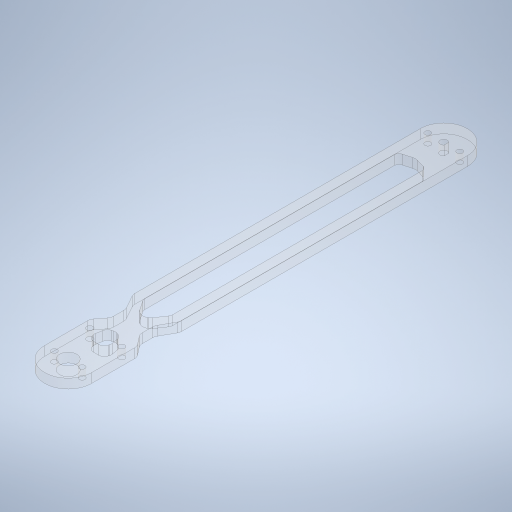
# Autodesk Inventor part: Part51
Saved by Autodesk Inventor 2024 (Build 280153000, 153)
## iProperties
Created: 2024-08-13
Part Number: Part51
Material: Polycarbonate, Clear
Document SubType Name: Modeling
Designer: David Ricaurte
Density: 1.2 g/cm^3
Appearance: Polycarbonate - Clear
Author: David Ricaurte
Autodesk Inventor part; units mm, degrees
ref_plane "YZ Plane" through (0, 0, 0) normal (1, 0, 0) x (0, 1, 0)
ref_plane "XZ Plane" through (0, 0, 0) normal (0, 1, 0) x (-1, 0, 0)
ref_plane "XY Plane" through (0, 0, 0) normal (0, 0, 1) x (1, 0, 0)
sketch "Sketch1" plane through (0, 0, 0) normal (0, 1, 0) x (-1, 0, 0)
  arc A0 (-1.4, -51.2845) -> (-1.4, -48.7155) centre (0, -50) ccw
  line L0 (-1.4, -48.7155) -> (-1.4, -51.2845)
  line L1 (-2.1842, 109.6159) -> (-1.9664, 109.7389)
  arc A1 (1.9664, 109.7389) -> (-1.9664, 109.7389) centre (0, 106.2556) ccw
  line L2 (1.9664, 109.7389) -> (2.1842, 109.6159)
  arc A2 (3.5277, 108.3788) -> (2.1842, 109.6159) centre (0.2179, 106.1326) ccw
  line L3 (3.5277, 108.3788) -> (8.2122, 101.4762)
  arc A3 (8.9023, 99.2105) -> (8.2122, 101.4762) centre (4.9024, 99.23) ccw
  line L4 (8.9023, 99.2105) -> (8.5178, 20.4265)
  arc A4 (5.6167, -33.4003) -> (8.5178, -29.5737) centre (4.5178, -29.5542) ccw
  line L5 (5.6167, -33.4003) -> (1.0989, -34.6911)
  arc A5 (-1.0989, -34.6911) -> (1.0989, -34.6911) centre (0, -30.845) ccw
  line L6 (-1.0989, -34.6911) -> (-5.6167, -33.4003)
  arc A6 (-8.5178, -29.5737) -> (-5.6167, -33.4003) centre (-4.5178, -29.5542) ccw
  line L7 (-8.5178, 20.4265) -> (-8.9023, 99.2105)
  arc A7 (-8.2122, 101.4762) -> (-8.9023, 99.2105) centre (-4.9024, 99.23) ccw
  line L8 (-8.2122, 101.4762) -> (-3.5277, 108.3788)
  arc A8 (-2.1842, 109.6159) -> (-3.5277, 108.3788) centre (-0.2179, 106.1326) ccw
  line L9 (-3.9333, 127.6797) -> (-4.4928, 131.0366)
  arc A9 (-4.4182, 132.354) -> (-4.4928, 131.0366) centre (-1.5336, 131.5298) ccw
  line L10 (-4.4182, 132.354) -> (-4.2433, 132.9662)
  arc A10 (-1.3587, 135.1421) -> (-4.2433, 132.9662) centre (-1.3587, 132.1421) ccw
  line L11 (-1.3587, 135.1421) -> (1.3587, 135.1421)
  arc A11 (4.2433, 132.9662) -> (1.3587, 135.1421) centre (1.3587, 132.1421) ccw
  line L12 (4.2433, 132.9662) -> (4.4182, 132.354)
  arc A12 (4.4928, 131.0366) -> (4.4182, 132.354) centre (1.5336, 131.5298) ccw
  line L13 (4.4928, 131.0366) -> (3.9333, 127.6797)
  arc A13 (1.7983, 125.2884) -> (3.9333, 127.6797) centre (0.9742, 128.1729) ccw
  line L14 (1.7983, 125.2884) -> (0.8242, 125.01)
  arc A14 (-0.8242, 125.01) -> (0.8242, 125.01) centre (0, 127.8946) ccw
  line L15 (-0.8242, 125.01) -> (-1.7983, 125.2884)
  arc A15 (-3.9333, 127.6797) -> (-1.7983, 125.2884) centre (-0.9742, 128.1729) ccw
  arc A16 (-12.5, 127.1805) -> (-11.6588, 124.7265) centre (-8.5, 127.1805) ccw
  line L16 (-11.6588, 124.7265) -> (-8.4827, 120.6384)
  arc A17 (-7.6415, 118.1843) -> (-8.4827, 120.6384) centre (-11.6415, 118.1843) ccw
  line L17 (-7.6415, 118.1843) -> (-7.6415, 112.7784)
  arc A18 (-8.147, 110.832) -> (-7.6415, 112.7784) centre (-11.6415, 112.7784) ccw
  line L18 (-8.147, 110.832) -> (-11.9945, 103.9244)
  arc A19 (-11.9945, 103.9244) -> (-12.5, 101.978) centre (-8.5, 101.978) ccw
  line L19 (-12.5, 101.978) -> (-12.5, 0)
  arc A20 (-12.5, -50) -> (12.5, -50) centre (0, -50) ccw
  line L20 (12.5, 0) -> (12.5, 101.978)
  arc A21 (12.5, 101.978) -> (11.9945, 103.9244) centre (8.5, 101.978) ccw
  line L21 (11.9945, 103.9244) -> (8.147, 110.832)
  arc A22 (7.6415, 112.7784) -> (8.147, 110.832) centre (11.6415, 112.7784) ccw
  line L22 (7.6415, 112.7784) -> (7.6415, 118.1843)
  arc A23 (8.4827, 120.6384) -> (7.6415, 118.1843) centre (11.6415, 118.1843) ccw
  line L23 (8.4827, 120.6384) -> (11.6588, 124.7265)
  arc A24 (11.6588, 124.7265) -> (12.5, 127.1805) centre (8.5, 127.1805) ccw
  line L24 (12.5, 127.1805) -> (12.5, 150)
  arc A25 (12.5, 150) -> (-12.5, 150) centre (0, 150) ccw
  line L25 (-12.5, 150) -> (-12.5, 127.1805)
  circle A26 centre (8.5, -50) radius 1.5
  circle A27 centre (-8.5, -50) radius 1.5
  circle A28 centre (0, 150) radius 4.5
  circle A29 centre (-8.5, 130) radius 1.6
  circle A30 centre (8.5, 130) radius 1.6
  circle A31 centre (-7.4, 150) radius 1.5
  circle A32 centre (7.4, 150) radius 1.5
  line L26 (0, 150) -> (0, -50)
  line L27 (0, -50) -> (0, -30.845)
  line L28 (12.5, 0) -> (12.5, -50)
  line L29 (-12.5, 0) -> (-12.5, -50)
  line L30 (-8.5178, 20.4265) -> (-8.5178, -29.5737)
  line L31 (8.5178, 20.4265) -> (8.5178, -29.5737)
  line L32 (7.4, 102.6729) -> (7.4, -32.3278)
  line L33 (-7.4, 102.6729) -> (-7.4, -32.3278)
  point P0 (0, 0)
  dimension "d0" = 200
  dimension "d1" = 19.155
  constraints: 68 end point, 53 point on circle, 33 centre point, 3 parallel, 3 vertical, 2 point on line, 2 symmetric about line
  measures "d0" distance of L26.start L26.end
  measures "d1" distance of L26.end L27.end
extrude "Extrusion1" add sketch "Sketch1" along normal blind 5 contours A6 L30 L7 A7 L8 L33 | L32 L3 A3 L4 L31 A4 | L25 A25 L24 A24 L23 A23 L22 A22 L21 A21 L20 L28 A20 L29 L19 A19 L18 A18 L17 A17 L16 A16
fillet "Fillet1" radius 2.5 4 edges at (7.4, 2.5, 102.6729) (-7.4, 2.5, 102.6729) (7.4, 2.5, -32.3278) (-7.4, 2.5, -32.3278)
body "Solid1"
